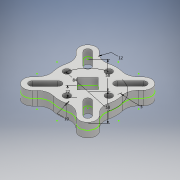
# Autodesk Inventor part: zad6.5-2
Saved by Autodesk Inventor 2018 (Build 220112000, 112)
## iProperties
Created: 2020-04-07
Part Number: zad6.5-2
Material: Типовые
Document SubType Name: Modeling
Designer: Аня
Density: 1 g/cm^3
Appearance: По умолчанию
Author: Аня
Autodesk Inventor part; units mm, degrees
ref_plane "YZ Plane" through (0, 0, 0) normal (1, 0, 0) x (0, 1, 0)
ref_plane "XZ Plane" through (0, 0, 0) normal (0, 1, 0) x (-1, 0, 0)
ref_plane "XY Plane" through (0, 0, 0) normal (0, 0, 1) x (1, 0, 0)
sketch "Эскиз1" plane through (0, 0, 0) normal (0, 0, 1) x (1, 0, 0)
  line L0 (-49.5613, 32.4789) -> (-46.1658, 29.0829)
  arc A0 (-9.9119, -41.0174) -> (-28.7247, -46.3187) centre (-14.5855, -60.4635) ccw
  arc A1 (-46.2454, -28.8817) -> (-40.9525, -10.0059) centre (-60.3846, -14.7369) ccw
  line L1 (-49.6779, -32.3128) -> (-46.2454, -28.8817)
  line L2 (-32.2026, -49.7951) -> (-28.7247, -46.3187)
  line L3 (32.4613, 49.4132) -> (29.0266, 45.9781)
  line L4 (32.5245, -49.8733) -> (29.0477, -46.396)
  arc A2 (-18.5358, -25.7178) -> (-25.5688, -18.634) centre (-21.8407, -21.9658) ccw
  line L5 (-44.4737, -37.5164) -> (-25.1681, -18.2338)
  line L6 (-37.4044, -44.5893) -> (-18.0882, -25.2701)
  arc A3 (-44.4737, -37.5164) -> (-37.4044, -44.5893) centre (-40.9402, -41.054) ccw
  arc A4 (49.4475, 32.4296) -> (32.4613, 49.4132) centre (40.9544, 40.9214) ccw
  arc A5 (40.6925, -10.0468) -> (46.2227, -29.1959) centre (60.1168, -14.8103) ccw
  arc A6 (40.6925, -10.0468) -> (40.6782, 10.0021) centre (-0.0661, -0.0514) ccw
  line L7 (49.7111, -32.6849) -> (46.2227, -29.1959)
  arc A7 (32.5245, -49.8733) -> (49.7111, -32.6849) centre (40.9242, -41.0855) ccw
  line L8 (-32.5896, 49.4483) -> (-29.1276, 45.9858)
  arc A8 (-29.1276, 45.9858) -> (-10.1722, 40.7146) centre (-14.9845, 60.1268) ccw
  arc A9 (-32.5896, 49.4483) -> (-49.5613, 32.4789) centre (-41.0754, 40.9636) ccw
  arc A10 (25.6897, -18.783) -> (18.5972, -25.7817) centre (21.8468, -21.9817) ccw
  line L9 (25.0502, -18.1426) -> (44.6422, -37.758)
  arc A11 (37.0996, -44.3062) -> (44.1505, -37.2657) centre (40.9242, -41.0855) ccw
  line L10 (18.043, -25.2269) -> (37.5945, -44.8016)
  arc A12 (45.9526, 28.9342) -> (40.6782, 10.0021) centre (60.0957, 14.7933) ccw
  line L11 (49.4475, 32.4296) -> (45.9526, 28.9342)
  arc A13 (-9.9119, -41.0174) -> (9.9867, -40.9672) centre (-0.0661, -0.0514) ccw
  line L12 (25.1074, 18.0466) -> (44.5086, 37.4248)
  arc A14 (44.2107, 37.1271) -> (37.4186, 44.4567) centre (40.9544, 40.9214) ccw
  line L13 (18.0631, 25.0983) -> (37.4186, 44.4567)
  arc A15 (-49.6779, -32.3128) -> (-32.2026, -49.7951) centre (-40.9402, -41.054) ccw
  arc A16 (-37.5378, 44.497) -> (-44.2965, 37.1394) centre (-41.0754, 40.9636) ccw
  arc A17 (-40.9011, 10.1117) -> (-46.1658, 29.0829) centre (-60.3089, 14.942) ccw
  line L14 (-25.2201, 18.0602) -> (-44.5957, 37.4386)
  line L15 (-37.5378, 44.497) -> (-18.1718, 25.108)
  arc A18 (-25.7906, 18.6308) -> (-18.7377, 25.6746) centre (-21.9811, 21.8692) ccw
  arc A19 (-40.9011, 10.1117) -> (-40.9525, -10.0059) centre (-0.0661, -0.0514) ccw
  arc A20 (10.0611, 40.7093) -> (-10.1722, 40.7146) centre (-0.0661, -0.0514) ccw
  arc A21 (18.6291, 25.6644) -> (25.6775, 18.616) centre (21.8705, 21.8574) ccw
  arc A22 (10.0611, 40.7093) -> (29.0266, 45.9781) centre (14.8836, 60.119) ccw
  arc A23 (29.0477, -46.396) -> (9.9867, -40.9672) centre (14.7586, -60.3893) ccw
  circle A24 centre (-30.9266, -0.0403) radius 5
  circle A25 centre (0.0734, -31.0403) radius 5
  circle A26 centre (31.0734, -0.0403) radius 5
  circle A27 centre (0.0734, 30.9597) radius 5
  line L16 (-0.2566, 15.4834) -> (15.4779, 0.1072)
  line L17 (15.4779, 0.1072) -> (0.1018, -15.6273)
  line L18 (0.1018, -15.6273) -> (-15.6327, -0.2511)
  line L19 (-15.6327, -0.2511) -> (-0.2566, 15.4834)
  point P0 (0, 0)
  dimension "d1" = 10
  dimension "d3" = 58
  dimension "d5" = 84
  dimension "d11" = 58
  dimension "d13" = 5
  dimension "d15" = 12
  dimension "d18" = 22
  constraints: 59 point on circle, 40 end point, 28 centre point, 25 tangent, 17 equal radius, 15 point on line, 12 parallel, 3 perpendicular
  measures "d1" diameter of A25
  measures "d3" distance of A6.centre A7.centre
  measures "d5" diameter of A20
  measures "d11" distance of A9.centre A6.centre
  measures "d13" radius of A21
  measures "d15" radius of A9
  measures "d18" distance of L17.end L18.end
sketch "Эскиз2" plane through (0, 0, 0) normal (0, 0, 1) x (1, 0, 0)
  point P0 (0, 0)
extrude "Выдавливание1" add sketch "Эскиз1" along normal blind 10
extrude "Выдавливание3" add sketch "Эскиз1" against normal blind 10
